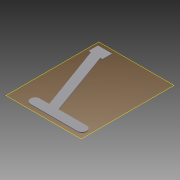
# Autodesk Inventor part: club_ABS_metal
Saved by Autodesk Inventor 2015 SP1 (Build 190203100, 203)
## iProperties
Created: 2015-03-24
Part Number: club_ABS_metal
Material: Ogólny
Document SubType Name: Konstrukcja blachowa
Designer: Marcin
Density: 1 g/cm^3
Sheet Metal Rule: Domyślny
Appearance: Domyślna
Author: Marcin
Autodesk Inventor part; units mm, degrees
ref_plane "YZ Plane" through (0, 0, 0) normal (1, 0, 0) x (0, 1, 0)
ref_plane "XZ Plane" through (0, 0, 0) normal (0, 1, 0) x (-1, 0, 0)
ref_plane "XY Plane" through (0, 0, 0) normal (0, 0, 1) x (1, 0, 0)
ref_plane "Płaszczyzna konstrukcyjna1" through (0, 0, 0) normal (0, 0, 1) x (1, 0, 0)
sketch "Szkic1" plane through (0, 0, 0) normal (0, 0, 1) x (1, 0, 0)
  line L0 (-7.6801, 0) -> (-5.1801, 0)
  line L1 (-5.1801, 0) -> (18.4779, -65)
  line L2 (18.4779, -65) -> (10.4779, -65)
  arc A0 (10.4779, -65) -> (10.4779, -85) centre (10.4779, -75) ccw
  line L3 (10.4779, -85) -> (80.4779, -85)
  arc A1 (80.4779, -85) -> (80.4779, -65) centre (80.4779, -75) ccw
  line L4 (80.4779, -65) -> (28.4779, -65)
  line L5 (28.4779, -65) -> (4.8199, 0)
  line L6 (4.8199, 0) -> (7.3199, 0)
  line L7 (7.3199, 0) -> (7.3199, 10)
  line L8 (7.3199, 10) -> (-7.6801, 10)
  line L9 (-7.6801, 10) -> (-7.6801, 0)
  point P0 (0, 0)
extrude "Płyta1" add sketch "Szkic1" along normal blind 0.8
equation "\"PromieńGięcia\" = Grubość"
equation "\"SzerokośćGięciaPodcięcia\" = Grubość"
equation "\"GłębokośćGięciaPodcięcia\" = 0.5 * Grubość"
equation "\"RozmiarPodcięciaNarożnika\" = 4 * Grubość"
equation "\"MinimalnaPozostałość\" = 2 * Grubość"
equation "\"PromieńPrzejścia\" = PromieńGięcia"
equation "\"Rozmiar_promienia_Jacobiego\" = Grubość"
equation "\"Wielk_odstępu\" = Grubość"
equation "\"d0\" = PromieńGięcia"
equation "\"Grubość\" = 0.8"
